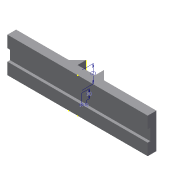
# Autodesk Inventor part: Tank Tread link A
Saved by Autodesk Inventor 2015 (Build 190159000, 159)
## iProperties
Created: 2015-03-14
Part Number: Tank Tread link A
Material: Generic
Document SubType Name: Modeling
Designer: james_000
Density: 1 g/cm^3
Appearance: Default
Author: james_000
Autodesk Inventor part; units mm, degrees
ref_plane "YZ Plane" through (0, 0, 0) normal (1, 0, 0) x (0, 1, 0)
ref_plane "XZ Plane" through (0, 0, 0) normal (0, 1, 0) x (-1, 0, 0)
ref_plane "XY Plane" through (0, 0, 0) normal (0, 0, 1) x (1, 0, 0)
sketch "Sketch1" plane through (0, 0, 0) normal (0, 0, 1) x (1, 0, 0)
  line L0 (-1, 2) -> (-2, 1)
  line L1 (1, 2) -> (2, 1)
  line L2 (-1, 2) -> (-1, 1)
  line L3 (-1, 1) -> (1, 1)
  line L4 (1, 1) -> (1, 2)
  line L5 (0, 0) -> (8, 0)
  line L6 (8, 0) -> (8, 1)
  line L7 (8, 1) -> (2, 1)
  line L8 (0, 0) -> (-8, 0)
  line L9 (-8, 0) -> (-8, 1)
  line L10 (-8, 1) -> (-2, 1)
  dimension "d7" = 2
  dimension "d8" = 1
  dimension "d9" = 2
  dimension "d29" = 8
  dimension "d30" = 8
  constraints: 22 end point, 6 perpendicular, 2 horizontal, 1 vertical
  measures "d7" distance of L0.start L1.start
  measures "d8" distance of L0.start L2.end
  measures "d9" distance of L2.end L3.end
  measures "d29" distance of L5.start L5.end
  measures "d30" distance of L5.start L8.end
extrude "Extrusion1" add sketch "Sketch1" along normal blind 4
sketch "Sketch2" plane through (-1, 1, 0) normal (1, 0, 0) x (0, 0, -1)
  line L0 (0, 0) -> (0, 1) projected
  line L1 (-4, 0) -> (-4, 1) projected
  circle A0 centre (-1, 0.5) radius 0.25
  circle A1 centre (-3, 0.5) radius 0.25
  point P0 (0, -1)
  dimension "d14" = 0.5
  dimension "d15" = 0.5
  constraints: 2 centre point
  measures "d14" diameter of A0
  measures "d15" diameter of A1
extrude "Extrusion2" add sketch "Sketch2" along normal blind 2 contours A0
sketch "Sketch3" plane through (-1, 1, 0) normal (1, 0, 0) x (0, 0, -1)
  line L0 (-4, 0) -> (-4, 1) projected
  circle A0 centre (-3, 0.5) radius 0.25
  point P0 (0, -1)
  dimension "d19" = 0.5
  constraints: 1 centre point
  measures "d19" diameter of A0
extrude "Extrusion3" add sketch "Sketch3" along normal blind 2
sketch "Sketch4" plane through (7, 0, 0) normal (1, 0, 0) x (0, 0, -1)
  line L0 (0, 0) -> (-1.3333, 0)
  line L1 (-1.3333, 0) -> (-1.3333, 0.3)
  line L2 (-1.3333, 0.3) -> (-2.6667, 0.3)
  line L3 (-2.6667, 0.3) -> (-2.6667, 0)
  point P0 (-4, 0)
  dimension "d22" = 1.3333
  dimension "d23" = 1.3333
  dimension "d24" = 0.3
  constraints: 8 end point, 2 perpendicular
  measures "d22" distance of point (-4, 0) L3.end
  measures "d23" distance of L0.start L0.end
  measures "d24" distance of L0.end L1.end
split "Split1" [suppressed]
sketch "Sketch5" plane through (-1, 1, 0) normal (1, 0, 0) x (0, 0, -1)
  line L0 (0, 0) -> (0, 1) projected
  circle A0 centre (-1, 0.5) radius 0.25 projected
  circle A1 centre (-3, 0.5) radius 0.25 projected
  point P0 (0, -1)
  dimension "d25" = 1
  dimension "d26" = 2
  measures "d25" distance from line of L0 A0.centre
  measures "d26" distance between centres of A1 A0
sketch "Sketch6" plane through (-1, 1, 0) normal (1, 0, 0) x (0, 0, -1)
  line L0 (0, 1) -> (-4, 1) projected
  circle A0 centre (-1, 0.5) radius 0.25 projected
  point P0 (0, -1)
  dimension "d27" = 0.5
  measures "d27" distance from line of L0 A0.centre
sketch "Sketch8" plane through (0, 0, 4) normal (0, 0, 1) x (1, 0, 0)
  point P0 (0, 0)
sketch "Sketch9" plane through (0, 0, 4) normal (0, 0, 1) x (1, 0, 0)
  point P0 (0, 0)
sketch "Sketch10" plane through (0, 0, 0) normal (0, 0, -1) x (-1, 0, 0)
  point P0 (0, 0)
sketch "Sketch11" plane through (-8, 0, 0) normal (-1, 0, 0) x (0, 0, 1)
  line L0 (2.6667, 0) -> (2.6667, 0.3)
  line L1 (2.6667, 0.3) -> (1.3333, 0.3)
  line L2 (1.3333, 0.3) -> (1.3333, 0)
  line L3 (2.6667, 0) -> (4, 0)
  point P0 (0, 0)
  dimension "d31" = 1.3333
  dimension "d32" = 1.3333
  dimension "d33" = 0.3
  constraints: 8 end point, 1 perpendicular, 1 vertical
  measures "d31" distance of point (0, 0) L2.end
  measures "d32" distance of L3.end L0.start
  measures "d33" distance of L0.start L0.end
split body "Split2" sketch "Sketch11" result one side removed curves L3 L0 L1 L2 removed pieces at (-2.6667, 0.1, 1.7778)
body "Solid1"
